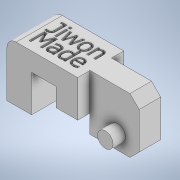
# Autodesk Inventor part: 14-1
Saved by Autodesk Inventor 2022 (Build 260153000, 153)
## iProperties
Created: 2021-09-12
Part Number: 14-1
Material: 일반
Document SubType Name: Modeling
Designer: 서울공업고등학교
Density: 1 g/cm^3
Appearance: 기본값
Author: 서울공업고등학교
Autodesk Inventor part; units mm, degrees
ref_plane "YZ Plane" through (0, 0, 0) normal (1, 0, 0) x (0, 1, 0)
ref_plane "XZ Plane" through (0, 0, 0) normal (0, 1, 0) x (-1, 0, 0)
ref_plane "XY Plane" through (0, 0, 0) normal (0, 0, 1) x (1, 0, 0)
sketch "스케치1" plane through (0, 0, 0) normal (0, 0, 1) x (1, 0, 0)
  circle A0 centre (0, 0) radius 2.5
  line L0 (-9, 13) -> (7, 13)
  line L1 (7, 13) -> (7, -5)
  line L2 (7, -5) -> (-9, -5)
  line L3 (-9, -5) -> (-9, 13)
  line L4 (-9, 13) -> (-32, 13)
  line L5 (-32, 13) -> (-32, -5)
  line L6 (-32, -5) -> (-24, -5)
  line L7 (-9, -5) -> (-9, 13)
  line L8 (-9, 1) -> (-16, 1)
  line L9 (-16, 1) -> (-16, 7)
  line L10 (-16, 7) -> (-24, 7)
  line L11 (-24, 7) -> (-24, 1)
  line L12 (-24, 1) -> (-24, -5)
  dimension "d0" = 16
  dimension "d1" = 18
  dimension "d2" = 5
  dimension "d3" = 7
  dimension "d4" = 13
  dimension "d5" = 39
  dimension "d6" = 6
  dimension "d7" = 12
  dimension "d8" = 8
  dimension "d9" = 23
  constraints: 26 end point, 6 perpendicular, 4 parallel, 3 point on line, 2 horizontal, 1 centre point, 1 coincident, 1 collinear
  measures "d0" distance of L1.end L2.end
  measures "d1" distance of L0.end L1.end
  measures "d2" diameter of A0
  measures "d3" distance from line of L1 point (0, 0)
  measures "d4" distance from line of L0 point (0, 0)
  measures "d5" distance between parallel lines of L1 L5
  measures "d6" distance between parallel lines of L6 L8
  measures "d7" distance between parallel lines of L6 L10
  measures "d8" distance between parallel lines of L11 L9
  measures "d9" distance between parallel lines of L1 L9
extrude "돌출1" add sketch "스케치1" along normal mid plane 15 contours L3 L8 L9 L10 L11 L12 L6 L5 L4
extrude "돌출2" add sketch "스케치1" along normal mid plane 7 contours A0 | L0 L1 L2 L3
extrude "돌출3" add sketch "스케치1" along normal mid plane 15 contours A0
chamfer "모따기1" distance 3 angle 45 1 edges at (7, 13, 0)
chamfer "모따기2" distance 3 angle 45 1 edges at (7, -5, 0)
fillet "모깎기1" radius 3 1 edges at (-32, 13, 0)
sketch "스케치2" plane through (-9, 13, 7.5) normal (0, 1, 0) x (1, 0, 0)
  line L0 (-18.8382, 13.0342) -> (2.851, 13.0342) construction
  line L1 (2.851, 13.0342) -> (2.851, 9.7862) construction
  line L2 (2.851, 9.7862) -> (-18.8382, 9.7862) construction
  line L3 (-18.8382, 9.7862) -> (-18.8382, 13.0342) construction
  spline S0 degree 2 poles (-16.4476, 9.3025) (-16.4476, 8.6461) (-17.2498, 7.9329) (-17.9265, 7.9329) knots 0 0 0 1 2 2 2
  spline S1 degree 2 poles (-17.9265, 7.9329) (-18.0886, 7.9329) (-18.6275, 7.9897) (-18.8098, 8.0302) knots 0 0 0 1 2 2 2
  line L4 (-18.8098, 8.0302) -> (-18.8098, 8.6704)
  line L5 (-18.8098, 8.6704) -> (-18.7733, 8.6704)
  spline S2 degree 2 poles (-18.7733, 8.6704) (-18.6356, 8.6218) (-18.2263, 8.5083) (-18.0156, 8.5083) knots 0 0 0 1 2 2 2
  spline S3 degree 2 poles (-18.0156, 8.5083) (-17.7077, 8.5083) (-17.339, 8.6501) (-17.2539, 8.7798) knots 0 0 0 1 2 2 2
  spline S4 degree 2 poles (-17.2539, 8.7798) (-17.1607, 8.9135) (-17.1121, 9.3025) (-17.1121, 9.5577) knots 0 0 0 1 2 2 2
  line L6 (-17.1121, 9.5577) -> (-17.1121, 12.471)
  line L7 (-17.1121, 12.471) -> (-18.1696, 12.471)
  line L8 (-18.1696, 12.471) -> (-18.1696, 13.0018)
  line L9 (-18.1696, 13.0018) -> (-16.4476, 13.0018)
  line L10 (-16.4476, 13.0018) -> (-16.4476, 9.3025)
  line L11 (-14.8714, 8.0018) -> (-15.5035, 8.0018)
  line L12 (-15.5035, 8.0018) -> (-15.5035, 11.7538)
  line L13 (-15.5035, 11.7538) -> (-14.8714, 11.7538)
  line L14 (-14.8714, 11.7538) -> (-14.8714, 8.0018)
  line L15 (-14.8268, 12.3778) -> (-15.544, 12.3778)
  line L16 (-15.544, 12.3778) -> (-15.544, 13.0342)
  line L17 (-15.544, 13.0342) -> (-14.8268, 13.0342)
  line L18 (-14.8268, 13.0342) -> (-14.8268, 12.3778)
  line L19 (-9.3973, 11.7538) -> (-10.3495, 8.0018)
  line L20 (-10.3495, 8.0018) -> (-10.933, 8.0018)
  line L21 (-10.933, 8.0018) -> (-11.8487, 10.8949)
  line L22 (-11.8487, 10.8949) -> (-12.7604, 8.0018)
  line L23 (-12.7604, 8.0018) -> (-13.3398, 8.0018)
  line L24 (-13.3398, 8.0018) -> (-14.3001, 11.7538)
  line L25 (-14.3001, 11.7538) -> (-13.6437, 11.7538)
  line L26 (-13.6437, 11.7538) -> (-12.9792, 8.8487)
  line L27 (-12.9792, 8.8487) -> (-12.0918, 11.7538)
  line L28 (-12.0918, 11.7538) -> (-11.5691, 11.7538)
  line L29 (-11.5691, 11.7538) -> (-10.6575, 8.8487)
  line L30 (-10.6575, 8.8487) -> (-10.0335, 11.7538)
  line L31 (-10.0335, 11.7538) -> (-9.3973, 11.7538)
  spline S5 degree 2 poles (-5.7588, 9.8778) (-5.7588, 8.9297) (-6.6704, 7.8965) (-7.4322, 7.8965) knots 0 0 0 1 2 2 2
  spline S6 degree 2 poles (-7.4322, 7.8965) (-8.2142, 7.8965) (-9.1096, 8.9621) (-9.1096, 9.8778) knots 0 0 0 1 2 2 2
  spline S7 degree 2 poles (-9.1096, 9.8778) (-9.1096, 10.8179) (-8.1858, 11.8592) (-7.4322, 11.8592) knots 0 0 0 1 2 2 2
  spline S8 degree 2 poles (-7.4322, 11.8592) (-6.6704, 11.8592) (-5.7588, 10.8219) (-5.7588, 9.8778) knots 0 0 0 1 2 2 2
  spline S9 degree 2 poles (-6.4111, 9.8778) (-6.4111, 10.6072) (-6.9419, 11.3162) (-7.4322, 11.3162) knots 0 0 0 1 2 2 2
  spline S10 degree 2 poles (-7.4322, 11.3162) (-7.9224, 11.3162) (-8.4573, 10.6072) (-8.4573, 9.8778) knots 0 0 0 1 2 2 2
  spline S11 degree 2 poles (-8.4573, 9.8778) (-8.4573, 9.1688) (-7.9224, 8.4394) (-7.4322, 8.4394) knots 0 0 0 1 2 2 2
  spline S12 degree 2 poles (-7.4322, 8.4394) (-6.9459, 8.4394) (-6.4111, 9.1566) (-6.4111, 9.8778) knots 0 0 0 1 2 2 2
  line L32 (-2.1647, 8.0018) -> (-2.7968, 8.0018)
  line L33 (-2.7968, 8.0018) -> (-2.7968, 10.1412)
  spline S13 degree 2 poles (-2.7968, 10.1412) (-2.7968, 10.4005) (-2.8455, 10.8462) (-2.9184, 10.9799) knots 0 0 0 1 2 2 2
  spline S14 degree 2 poles (-2.9184, 10.9799) (-2.9954, 11.1218) (-3.2709, 11.2595) (-3.5059, 11.2595) knots 0 0 0 1 2 2 2
  spline S15 degree 2 poles (-3.5059, 11.2595) (-3.7409, 11.2595) (-4.2393, 11.0083) (-4.4784, 10.8057) knots 0 0 0 1 2 2 2
  line L34 (-4.4784, 10.8057) -> (-4.4784, 8.0018)
  line L35 (-4.4784, 8.0018) -> (-5.1105, 8.0018)
  line L36 (-5.1105, 8.0018) -> (-5.1105, 11.7538)
  line L37 (-5.1105, 11.7538) -> (-4.4784, 11.7538)
  line L38 (-4.4784, 11.7538) -> (-4.4784, 11.3365)
  spline S16 degree 2 poles (-4.4784, 11.3365) (-4.1947, 11.5918) (-3.6477, 11.8592) (-3.3398, 11.8592) knots 0 0 0 1 2 2 2
  spline S17 degree 2 poles (-3.3398, 11.8592) (-2.7887, 11.8592) (-2.1647, 11.1299) (-2.1647, 10.437) knots 0 0 0 1 2 2 2
  line L39 (-2.1647, 10.437) -> (-2.1647, 8.0018)
  line L40 (-14.0448, 2.5018) -> (-14.7093, 2.5018)
  line L41 (-14.7093, 2.5018) -> (-14.7093, 6.809)
  line L42 (-14.7093, 6.809) -> (-16.014, 3.8795)
  line L43 (-16.014, 3.8795) -> (-16.4192, 3.8795)
  line L44 (-16.4192, 3.8795) -> (-17.7118, 6.809)
  line L45 (-17.7118, 6.809) -> (-17.7118, 2.5018)
  line L46 (-17.7118, 2.5018) -> (-18.3317, 2.5018)
  line L47 (-18.3317, 2.5018) -> (-18.3317, 7.5018)
  line L48 (-18.3317, 7.5018) -> (-17.4241, 7.5018)
  line L49 (-17.4241, 7.5018) -> (-16.1761, 4.7182)
  line L50 (-16.1761, 4.7182) -> (-14.9686, 7.5018)
  line L51 (-14.9686, 7.5018) -> (-14.0448, 7.5018)
  line L52 (-14.0448, 7.5018) -> (-14.0448, 2.5018)
  spline S18 degree 2 poles (-10.9897, 2.8989) (-11.0667, 2.8422) (-11.326, 2.6396) (-11.4476, 2.5788) knots 0 0 0 1 2 2 2
  spline S19 degree 2 poles (-11.4476, 2.5788) (-11.6137, 2.4897) (-11.9257, 2.3965) (-12.2093, 2.3965) knots 0 0 0 1 2 2 2
  spline S20 degree 2 poles (-12.2093, 2.3965) (-12.4403, 2.3965) (-12.8576, 2.5707) (-13.0156, 2.7287) knots 0 0 0 1 2 2 2
  spline S21 degree 2 poles (-13.0156, 2.7287) (-13.1656, 2.8827) (-13.3479, 3.3365) (-13.3479, 3.5877) knots 0 0 0 1 2 2 2
  spline S22 degree 2 poles (-13.3479, 3.5877) (-13.3479, 3.9767) (-13.0197, 4.5278) (-12.6631, 4.6858) knots 0 0 0 1 2 2 2
  spline S23 degree 2 poles (-12.6631, 4.6858) (-12.3471, 4.8316) (-11.4881, 4.941) (-10.9897, 4.9694) knots 0 0 0 1 2 2 2
  line L53 (-10.9897, 4.9694) -> (-10.9897, 5.091)
  spline S24 degree 2 poles (-10.9897, 5.091) (-10.9897, 5.3098) (-11.1234, 5.5812) (-11.245, 5.6582) knots 0 0 0 1 2 2 2
  spline S25 degree 2 poles (-11.245, 5.6582) (-11.3665, 5.7352) (-11.715, 5.7838) (-11.9014, 5.7838) knots 0 0 0 1 2 2 2
  spline S26 degree 2 poles (-11.9014, 5.7838) (-12.1202, 5.7838) (-12.7118, 5.6542) (-13.0075, 5.5286) knots 0 0 0 1 2 2 2
  line L54 (-13.0075, 5.5286) -> (-13.044, 5.5286)
  line L55 (-13.044, 5.5286) -> (-13.044, 6.1728)
  spline S27 degree 2 poles (-13.044, 6.1728) (-12.8698, 6.2214) (-12.2174, 6.343) (-11.8973, 6.343) knots 0 0 0 1 2 2 2
  spline S28 degree 2 poles (-11.8973, 6.343) (-11.5083, 6.343) (-10.9776, 6.2214) (-10.7669, 6.0634) knots 0 0 0 1 2 2 2
  spline S29 degree 2 poles (-10.7669, 6.0634) (-10.5602, 5.9094) (-10.3576, 5.4192) (-10.3576, 5.0667) knots 0 0 0 1 2 2 2
  line L56 (-10.3576, 5.0667) -> (-10.3576, 2.5018)
  line L57 (-10.3576, 2.5018) -> (-10.9897, 2.5018)
  line L58 (-10.9897, 2.5018) -> (-10.9897, 2.8989)
  line L59 (-10.9897, 3.4256) -> (-10.9897, 4.467)
  spline S30 degree 2 poles (-10.9897, 4.467) (-11.2166, 4.4467) (-11.9014, 4.3778) (-12.1161, 4.313) knots 0 0 0 1 2 2 2
  spline S31 degree 2 poles (-12.1161, 4.313) (-12.3673, 4.236) (-12.6955, 3.9159) (-12.6955, 3.6323) knots 0 0 0 1 2 2 2
  spline S32 degree 2 poles (-12.6955, 3.6323) (-12.6955, 3.3081) (-12.3309, 2.9799) (-11.9824, 2.9799) knots 0 0 0 1 2 2 2
  spline S33 degree 2 poles (-11.9824, 2.9799) (-11.6866, 2.9799) (-11.2004, 3.2352) (-10.9897, 3.4256) knots 0 0 0 1 2 2 2
  line L60 (-6.5853, 2.5018) -> (-7.2174, 2.5018)
  line L61 (-7.2174, 2.5018) -> (-7.2174, 2.8827)
  spline S34 degree 2 poles (-7.2174, 2.8827) (-7.3633, 2.7611) (-7.578, 2.5991) (-7.7239, 2.5302) knots 0 0 0 1 2 2 2
  spline S35 degree 2 poles (-7.7239, 2.5302) (-7.8576, 2.4654) (-8.1453, 2.3965) (-8.3357, 2.3965) knots 0 0 0 1 2 2 2
  spline S36 degree 2 poles (-8.3357, 2.3965) (-8.6437, 2.3965) (-9.1623, 2.6517) (-9.3447, 2.8989) knots 0 0 0 1 2 2 2
  spline S37 degree 2 poles (-9.3447, 2.8989) (-9.527, 3.1461) (-9.7296, 3.8754) (-9.7296, 4.3495) knots 0 0 0 1 2 2 2
  spline S38 degree 2 poles (-9.7296, 4.3495) (-9.7296, 4.8438) (-9.4743, 5.565) (-9.2515, 5.8365) knots 0 0 0 1 2 2 2
  spline S39 degree 2 poles (-9.2515, 5.8365) (-9.0448, 6.0796) (-8.4654, 6.3592) (-8.1453, 6.3592) knots 0 0 0 1 2 2 2
  spline S40 degree 2 poles (-8.1453, 6.3592) (-7.8657, 6.3592) (-7.4484, 6.2336) (-7.2174, 6.1039) knots 0 0 0 1 2 2 2
  line L62 (-7.2174, 6.1039) -> (-7.2174, 7.7247)
  line L63 (-7.2174, 7.7247) -> (-6.5853, 7.7247)
  line L64 (-6.5853, 7.7247) -> (-6.5853, 2.5018)
  line L65 (-7.2174, 3.4135) -> (-7.2174, 5.5812)
  spline S41 degree 2 poles (-7.2174, 5.5812) (-7.4524, 5.6947) (-7.8252, 5.7798) (-8.04, 5.7798) knots 0 0 0 1 2 2 2
  spline S42 degree 2 poles (-8.04, 5.7798) (-8.5262, 5.7798) (-9.0772, 5.0504) (-9.0772, 4.3616) knots 0 0 0 1 2 2 2
  spline S43 degree 2 poles (-9.0772, 4.3616) (-9.0772, 3.6971) (-8.6558, 2.9961) (-8.1899, 2.9961) knots 0 0 0 1 2 2 2
  spline S44 degree 2 poles (-8.1899, 2.9961) (-7.9427, 2.9961) (-7.4403, 3.2231) (-7.2174, 3.4135) knots 0 0 0 1 2 2 2
  spline S45 degree 2 poles (-4.0408, 2.4167) (-4.9403, 2.4167) (-5.9289, 3.4256) (-5.9289, 4.3576) knots 0 0 0 1 2 2 2
  spline S46 degree 2 poles (-5.9289, 4.3576) (-5.9289, 5.2733) (-4.9686, 6.3592) (-4.1947, 6.3592) knots 0 0 0 1 2 2 2
  spline S47 degree 2 poles (-4.1947, 6.3592) (-3.8463, 6.3592) (-3.3074, 6.1566) (-3.1088, 5.9419) knots 0 0 0 1 2 2 2
  spline S48 degree 2 poles (-3.1088, 5.9419) (-2.9062, 5.7271) (-2.6915, 5.1072) (-2.6915, 4.6574) knots 0 0 0 1 2 2 2
  line L66 (-2.6915, 4.6574) -> (-2.6915, 4.313)
  line L67 (-2.6915, 4.313) -> (-5.2887, 4.313)
  spline S49 degree 2 poles (-5.2887, 4.313) (-5.2887, 3.6607) (-4.6323, 2.9678) (-4.0489, 2.9678) knots 0 0 0 1 2 2 2
  spline S50 degree 2 poles (-4.0489, 2.9678) (-3.8422, 2.9678) (-3.4411, 3.061) (-3.279, 3.1339) knots 0 0 0 1 2 2 2
  spline S51 degree 2 poles (-3.279, 3.1339) (-3.1088, 3.215) (-2.8738, 3.3568) (-2.7968, 3.4216) knots 0 0 0 1 2 2 2
  line L68 (-2.7968, 3.4216) -> (-2.7604, 3.4216)
  line L69 (-2.7604, 3.4216) -> (-2.7604, 2.7328)
  spline S52 degree 2 poles (-2.7604, 2.7328) (-2.8698, 2.6882) (-3.202, 2.5585) (-3.3317, 2.5221) knots 0 0 0 1 2 2 2
  spline S53 degree 2 poles (-3.3317, 2.5221) (-3.514, 2.4694) (-3.8139, 2.4167) (-4.0408, 2.4167) knots 0 0 0 1 2 2 2
  spline S54 degree 2 poles (-3.3074, 4.7952) (-3.3155, 5.0504) (-3.4208, 5.4232) (-3.5221, 5.5488) knots 0 0 0 1 2 2 2
  spline S55 degree 2 poles (-3.5221, 5.5488) (-3.6315, 5.6906) (-3.9759, 5.8406) (-4.2312, 5.8406) knots 0 0 0 1 2 2 2
  spline S56 degree 2 poles (-4.2312, 5.8406) (-4.4824, 5.8406) (-4.8349, 5.6906) (-4.9808, 5.5448) knots 0 0 0 1 2 2 2
  spline S57 degree 2 poles (-4.9808, 5.5448) (-5.1226, 5.3949) (-5.2685, 5.0342) (-5.2887, 4.7952) knots 0 0 0 1 2 2 2
  line L70 (-5.2887, 4.7952) -> (-3.3074, 4.7952)
  point P0 (9, 7.5)
  constraints: 2 other
extrude "돌출4" cut sketch "스케치2" against normal blind 1
